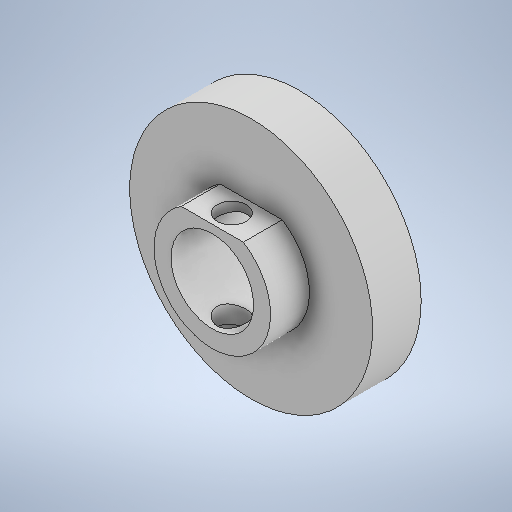
# Autodesk Inventor part: Project_Stationary_Wheel[1]
Saved by Autodesk Inventor 2025.1 (Build 291241020, 241B)
## iProperties
Created: 2025-09-02
Part Number: Project_Stationary_Wheel[1]
Material: Generic
Document SubType Name: Modeling
Designer: Kiran
Density: 1 g/cm^3
Appearance: Default
Author: Kiran
Autodesk Inventor part; units mm, degrees
ref_plane "YZ Plane" through (0, 0, 0) normal (1, 0, 0) x (0, 1, 0)
ref_plane "XZ Plane" through (0, 0, 0) normal (0, 1, 0) x (-1, 0, 0)
ref_plane "XY Plane" through (0, 0, 0) normal (0, 0, 1) x (1, 0, 0)
sketch "Sketch3" plane through (0, 0, 0) normal (0, 0, 1) x (1, 0, 0)
  circle A0 centre (0, 0) radius 25
  circle A1 centre (0, 0) radius 8.5
  dimension "d8" = 50
  dimension "d16" = 17
  constraints: 2 centre point, 2 coincident
  measures "d8" diameter of A0
  measures "d16" diameter of A1
extrude "Extrusion3" add sketch "Sketch3" along normal blind 10 contours A0 | A1
sketch "Sketch4" plane through (0, 0, 10) normal (0, 0, 1) x (1, 0, 0)
  circle A0 centre (0, 0) radius 12
  circle A1 centre (0, 0) radius 8.5
  dimension "d12" = 24
  dimension "d17" = 17
  constraints: 2 centre point, 2 coincident
  measures "d12" diameter of A0
  measures "d17" diameter of A1
extrude "Extrusion4" add sketch "Sketch4" along normal blind 8 contours A0 | A1
sketch "Sketch5" plane through (0, 0, 10) normal (0, 0, 1) x (1, 0, 0)
  point P0 (0, 0)
sketch "Sketch6" plane through (0, 0, 18) normal (0, 0, 1) x (1, 0, 0)
  circle A0 centre (0, 0) radius 8.5
  dimension "d18" = 17
  constraints: 1 centre point, 1 coincident
  measures "d18" diameter of A0
extrude "Extrusion5" cut sketch "Sketch6" against normal blind 30
sketch "Sketch7" plane through (0, 0, 18) normal (0, 0, 1) x (1, 0, 0)
  circle A0 centre (0, 0) radius 12 projected
  line L0 (6.3883, 10.1583) -> (-6.3883, 10.1583)
  arc A1 (6.3883, 10.1583) -> (-6.3883, 10.1583) centre (0, 0) ccw
  arc A2 (6.3883, 10.1583) -> (-6.3883, 10.1583) centre (0, 0) ccw
  constraints: 6 point on circle, 2 centre point, 2 coincident, 2 end point, 1 horizontal
extrude "Extrusion6" cut sketch "Sketch7" against normal blind 8 contours L0 A0 picked at (-1.322, 10.5474)
sketch "Sketch8" plane through (-6.3883, 10.1583, 18) normal (0, 1, 0) x (1, 0, 0)
  point P0 (6.3883, 18)
  point P1 (6.3883, 4)
hole "Hole1" at (0, 10.1583, 14) direction (0, -1, 0) diameter 6 end through all
body "Solid2"
